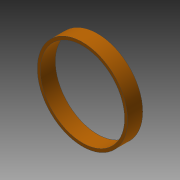
# Autodesk Inventor part: Tread
Saved by Autodesk Inventor 2014 (Build 180170000, 170)
## iProperties
Created: 2014-01-08
Part Number: Tread
Material: ABS Plastic
Document SubType Name: Modeling
Designer: Kelby
Mass: 63.3016 g
Surface Area: 282.135 cm^2
Volume: 59.7185 cm^3
Density: 1.06 g/cm^3
Appearance: Smooth - White
Author: Kelby
Autodesk Inventor part; units mm, degrees
ref_plane "YZ Plane" through (0, 0, 0) normal (1, 0, 0) x (0, 1, 0)
ref_plane "XZ Plane" through (0, 0, 0) normal (0, 1, 0) x (-1, 0, 0)
ref_plane "XY Plane" through (0, 0, 0) normal (0, 0, 1) x (1, 0, 0)
sketch "Sketch1" plane through (0, 0, 0) normal (0, 0, 1) x (1, 0, 0)
  circle A0 centre (0, -71.12) radius 12.7 construction
  circle A1 centre (0, -71.12) radius 76.2
  circle A2 centre (0, -71.12) radius 71.12 projected
  point P0 (0, 0)
  dimension "d0" = 152.4
  constraints: 1 centre point, 1 coincident
  measures "d0" diameter of A1
extrude "Extrusion1" add sketch "Sketch1" along normal blind 25.4
body "Solid1"
